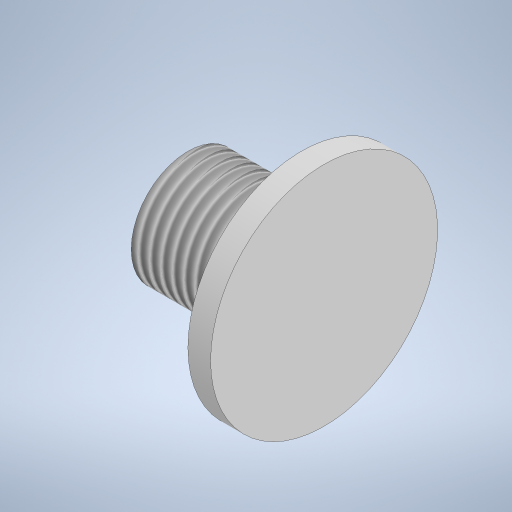
# Autodesk Inventor part: Болт маховика
Saved by Autodesk Inventor 2023 (Build 270158000, 158)
## iProperties
Created: 2022-05-01
Part Number: Болт маховика
Material: Типовые
Document SubType Name: Modeling
Designer: User
Density: 1 g/cm^3
Appearance: По умолчанию
Author: User
Autodesk Inventor part; units mm, degrees
ref_plane "YZ Plane" through (0, 0, 0) normal (1, 0, 0) x (0, 1, 0)
ref_plane "XZ Plane" through (0, 0, 0) normal (0, 1, 0) x (-1, 0, 0)
ref_plane "XY Plane" through (0, 0, 0) normal (0, 0, 1) x (1, 0, 0)
sketch "Эскиз1" plane through (0, 0, 0) normal (0, 1, 0) x (-1, 0, 0)
  line L0 (0, 0) -> (0, 15)
  line L1 (0, 15) -> (3, 15)
  line L2 (0, 0) -> (3, 0)
  line L3 (3, 0) -> (18, 0)
  line L4 (18, 0) -> (18, 7.5)
  line L5 (18, 7.5) -> (6, 7.5)
  line L6 (3, 7.5) -> (3, 15)
  line L7 (3, 15) -> (3, 8)
  line L8 (3, 8) -> (6, 8)
  line L9 (6, 8) -> (6, 7.5)
  dimension "d0" = 15
  dimension "d1" = 3
  dimension "d2" = 15
  dimension "d3" = 7.5
  dimension "d4" = 7
  dimension "d5" = 3
  constraints: 20 end point, 6 perpendicular, 2 point on line, 1 horizontal, 1 vertical
  measures "d0" distance of L0.start L0.end
  measures "d1" distance of L0.end L1.end
  measures "d2" distance of L2.end L3.end
  measures "d3" distance of L3.end L4.end
  measures "d4" distance of L1.end L7.end
  measures "d5" distance of L7.end L8.end
revolve "Вращение1" add sketch "Эскиз1" angle 360 about axis through (-3, 0, 0) along (-1, 0, 0)
thread "Резьба1" size "M15x1.5" class "6g" standard "ISO Metric profile" full length
